BasicRing v3 (Autodesk Fusion 360 design; units mm, degrees)
Autodesk Fusion 360 part; units mm, degrees
sketch "Sketch2" plane through (0, 0, 0) normal (0, 1, 0) x (1, 0, 0)
  circle A0 centre (0, 0) radius 45
  circle A1 centre (0, 0) radius 37
  dimension "d3" = 90
  dimension "d7" = -8
  constraint coincident A0.centre A1.centre
  measures "d3" diameter of A0
extrude "Extrude1" add sketch "Sketch2" along normal mid plane 3
sketch "Sketch1" plane through (0, 1.5, 0) normal (0, 1, 0) x (1, 0, 0)
  circle A0 centre (0, 41) radius 3.275
  circle A1 centre (0, 0) radius 37
  circle A2 centre (0, 0) radius 45
  line L0 (0, 45) -> (0, 41) construction
  line L1 (0, 41) -> (0, 37) construction
  dimension "d2" = 6.55
  constraint coincident A2 L0.start
  constraint coincident A0.centre L0.end
  constraint coincident A1 L1.end
  constraint equal L0 L1
  constraint collinear L0 L1
  constraint collinear A1.centre A0.centre L1.end
  constraint vertical L0
  measures "d2" diameter of A0
extrude "Extrude2" cut sketch "Sketch1" against normal through all contours A0
chamfer "Chamfer1" distance 0.2 angle 70 1 edges at (-3.0534, 1.5, -42.1843) measured on face at (42.028, 1.5, 4.0738)
pattern_circular "C-Pattern1" count 3 over 360 about axis through (0, 1.5, 0) along (0, -1, 0) of "Extrude2", "Chamfer1"
fillet "Fillet1" radius 0.5 2 edges at (-41.9547, 1.5, 16.2727) (-34.4961, 1.5, -13.3798)
equation "dowell_offset = 0.1 mm"
equation "d2 = dowell_diameter + ( 2 * dowell_offset )"
equation "d3 = ( 45 * 2 ) * 1 mm"
equation "dowell_diameter = ( 1 in / 4 in ) * 1 in"
